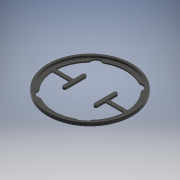
# Autodesk Inventor part: bumper_modified2
Saved by Autodesk Inventor 2017 SP1 (Build 210196100, 196)
## iProperties
Created: 2016-07-25
Part Number: bumper_modified2
Material: Plastique ABS
Document SubType Name: Modeling
Designer: tmonglon
Density: 1.06 g/cm^3
Appearance: Lisse - Noir
Author: tmonglon
Autodesk Inventor part; units mm, degrees
ref_plane "YZ Plane" through (0, 0, 0) normal (1, 0, 0) x (0, 1, 0)
ref_plane "XZ Plane" through (0, 0, 0) normal (0, 1, 0) x (-1, 0, 0)
ref_plane "XY Plane" through (0, 0, 0) normal (0, 0, 1) x (1, 0, 0)
sketch "Esquisse1" plane through (0, 0, 0) normal (0, 0, 1) x (1, 0, 0)
  circle A0 centre (0, 0) radius 63
  circle A1 centre (0, 0) radius 60
  circle A2 centre (0, 0) radius 54
  line L0 (-25.9421, 2.5) -> (-53.9421, 2.5)
  line L1 (-25.9421, -2.5) -> (-53.9421, -2.5)
  line L2 (-20.9421, 0) -> (-20.9421, 14.5)
  line L3 (-25.9421, 14.5) -> (-25.9421, 2.5)
  line L4 (-20.9421, 0) -> (-20.9421, -14.5)
  line L5 (-25.9421, -14.5) -> (-25.9421, 2.5)
  arc A3 (-25.9421, -14.5) -> (-20.9421, -14.5) centre (-23.4421, -14.5) ccw
  arc A4 (-20.9421, 14.5) -> (-25.9421, 14.5) centre (-23.4421, 14.5) ccw
  line L6 (0, 0) -> (0, 11.8583)
  line L7 (25.9421, 2.5) -> (53.9421, 2.5)
  line L8 (25.9421, -2.5) -> (53.9421, -2.5)
  line L9 (20.9421, 0) -> (20.9421, 14.5)
  line L10 (25.9421, 14.5) -> (25.9421, 2.5)
  line L11 (20.9421, 0) -> (20.9421, -14.5)
  line L12 (25.9421, -14.5) -> (25.9421, 14.5)
  arc A5 (20.9421, -14.5) -> (25.9421, -14.5) centre (23.4421, -14.5) ccw
  arc A6 (25.9421, 14.5) -> (20.9421, 14.5) centre (23.4421, 14.5) ccw
  line L13 (25.9421, 2.5) -> (56.5559, 2.5)
  line L14 (56.5559, 2.5) -> (56.5559, -2.5)
  line L15 (56.5559, -2.5) -> (25.9421, -2.5)
  line L16 (25.9421, -2.5) -> (25.9421, 2.5)
  dimension "d0" = 126
  dimension "d1" = 120
  dimension "d2" = 108
  dimension "d3" = 28
  dimension "d6" = 14.5
  dimension "d8" = 5
  constraints: 34 end point, 11 point on circle, 11 symmetric about line, 7 centre point, 6 point on line, 4 parallel, 1 coincident, 1 horizontal, 1 perpendicular, 1 vertical, 2 other
  measures "d0" diameter of A0
  measures "d1" diameter of A1
  measures "d2" diameter of A2
  measures "d3" distance of L0.start L0.end
  measures "d6" distance of L2.start L2.end
  measures "d8" distance of L4.end L5.start
extrude "Extrusion1" add sketch "Esquisse1" along normal blind 5 contours A0
extrude "Extrusion2" add sketch "Esquisse1" along normal blind 1.7 contours A1 | A2 L8 L12 L7 | A2 L13 L14 L15 | L0 L5 L1 A2
sketch "Esquisse3" plane through (0, 0, 0) normal (0, 0, -1) x (-1, 0, 0)
  line L0 (20.9421, 0) -> (20.9421, 14.5) projected
  line L1 (20.9421, 0) -> (20.9421, -14.5) projected
  arc A0 (20.9421, -14.5) -> (25.9421, -14.5) centre (23.4421, -14.5) ccw projected
  line L2 (25.9421, -14.5) -> (25.9421, 2.5) projected
  line L3 (25.9421, 14.5) -> (25.9421, 2.5) projected
  arc A1 (25.9421, 14.5) -> (20.9421, 14.5) centre (23.4421, 14.5) ccw projected
  arc A2 (-20.9421, 14.5) -> (-25.9421, 14.5) centre (-23.4421, 14.5) ccw projected
  line L4 (-25.9421, 14.5) -> (-25.9421, 2.5) projected
  line L5 (-25.9421, -14.5) -> (-25.9421, 14.5) projected
  arc A3 (-25.9421, -14.5) -> (-20.9421, -14.5) centre (-23.4421, -14.5) ccw projected
  line L6 (-20.9421, 0) -> (-20.9421, -14.5) projected
  line L7 (-20.9421, 0) -> (-20.9421, 14.5) projected
  point P0 (0, 0)
extrude "Extrusion3" add sketch "Esquisse3" against normal blind 3
fillet "Congé1" radius 1 3 edges at (25.9421, 0, 1.7) (25.9421, -2.5, 0.85) (25.9421, 2.5, 0.85)
fillet "Congé2" radius 1 3 edges at (-25.9421, 0, 1.7) (-25.9421, -2.5, 0.85) (-25.9421, 2.5, 0.85)
fillet "Congé3" radius 1 4 edges at (53.9421, 2.5, 0.85) (53.9421, -2.5, 0.85) (-53.9421, 2.5, 0.85) (-53.9421, -2.5, 0.85)
sketch "Esquisse4" plane through (0, 0, 0) normal (0, 0, -1) x (-1, 0, 0)
  arc A0 (53.8821, 3.566) -> (-53.8821, 3.566) centre (0, 0) ccw projected
  arc A1 (-53.8821, -3.566) -> (53.8821, -3.566) centre (0, 0) ccw projected
  arc A2 (53.8821, 3.566) -> (-53.8821, 3.566) centre (0, 0) ccw projected
  arc A3 (52.8843, 2.5) -> (53.8821, 3.566) centre (52.8843, 3.5) ccw projected
  line L0 (52.8843, 2.5) -> (26.9421, 2.5) projected
  arc A4 (25.9421, 3.5) -> (26.9421, 2.5) centre (26.9421, 3.5) ccw projected
  line L1 (25.9421, 3.5) -> (25.9421, 14.5) projected
  arc A5 (25.9421, 14.5) -> (20.9421, 14.5) centre (23.4421, 14.5) ccw projected
  line L2 (20.9421, 14.5) -> (20.9421, -14.5) projected
  arc A6 (20.9421, -14.5) -> (25.9421, -14.5) centre (23.4421, -14.5) ccw projected
  line L3 (25.9421, -14.5) -> (25.9421, -3.5) projected
  arc A7 (26.9421, -2.5) -> (25.9421, -3.5) centre (26.9421, -3.5) ccw projected
  line L4 (26.9421, -2.5) -> (52.8843, -2.5) projected
  arc A8 (53.8821, -3.566) -> (52.8843, -2.5) centre (52.8843, -3.5) ccw projected
  arc A9 (-53.8821, -3.566) -> (53.8821, -3.566) centre (0, 0) ccw projected
  arc A10 (-52.8843, -2.5) -> (-53.8821, -3.566) centre (-52.8843, -3.5) ccw projected
  line L5 (-26.9421, -2.5) -> (-52.8843, -2.5) projected
  arc A11 (-25.9421, -3.5) -> (-26.9421, -2.5) centre (-26.9421, -3.5) ccw projected
  line L6 (-25.9421, -3.5) -> (-25.9421, -14.5) projected
  arc A12 (-25.9421, -14.5) -> (-20.9421, -14.5) centre (-23.4421, -14.5) ccw projected
  line L7 (-20.9421, -14.5) -> (-20.9421, 14.5) projected
  arc A13 (-20.9421, 14.5) -> (-25.9421, 14.5) centre (-23.4421, 14.5) ccw projected
  line L8 (-25.9421, 14.5) -> (-25.9421, 3.5) projected
  arc A14 (-26.9421, 2.5) -> (-25.9421, 3.5) centre (-26.9421, 3.5) ccw projected
  line L9 (-52.8843, 2.5) -> (-26.9421, 2.5) projected
  arc A15 (-53.8821, 3.566) -> (-52.8843, 2.5) centre (-52.8843, 3.5) ccw projected
  circle A16 centre (0, 0) radius 63 projected
  line L10 (32.9786, 41.9728) -> (-33, 41.9728)
  line L11 (-33, 41.9728) -> (-33, -42)
  line L12 (-33, -42) -> (32.9786, -42)
  line L13 (32.9786, -42) -> (32.9786, 41.9728)
  line L14 (32.9786, 32.8) -> (-33, 32.8)
  line L15 (32.9786, -32.8) -> (-33, -32.8)
  line L16 (-33.3624, -42.4612) -> (38.9228, 49.5381)
  line L17 (33.3492, -42.4716) -> (-38.936, 49.5277)
  line L18 (-33.2831, 42.3332) -> (-36.4284, 39.8619)
  line L19 (-33.2831, 42.3332) -> (-30.1379, 44.8045)
  arc A17 (-30.1379, 44.8045) -> (-36.4284, 39.8619) centre (-32.5624, 41.4158) ccw
  line L20 (33.2707, 42.3445) -> (30.1254, 44.8158)
  line L21 (33.2707, 42.3445) -> (36.416, 39.8733)
  line L22 (33.2831, -42.3332) -> (36.4284, -39.8619)
  line L23 (33.2831, -42.3332) -> (30.1379, -44.8045)
  arc A18 (30.1379, -44.8045) -> (36.4284, -39.8619) centre (32.5624, -41.4158) ccw
  arc A19 (36.416, 39.8733) -> (30.1254, 44.8158) centre (32.5499, 41.4272) ccw
  line L24 (-33.2707, -42.3445) -> (-36.416, -39.8733)
  arc A20 (-36.416, -39.8733) -> (-30.1254, -44.8158) centre (-32.5499, -41.4272) ccw
  line L25 (-33.2707, -42.3445) -> (-30.1254, -44.8158)
  arc A21 (-53.8821, -3.566) -> (53.8821, -3.566) centre (0, 0) ccw projected
  line L26 (-38.5851, -37.7782) -> (-27.5766, -46.4277)
  arc A22 (-38.5851, -37.7782) -> (-27.5766, -46.4277) centre (-31.4173, -39.9857) ccw
  line L27 (-38.5969, 37.7661) -> (-27.5885, 46.4156)
  arc A23 (-27.5885, 46.4156) -> (-38.5969, 37.7661) centre (-31.4292, 39.9736) ccw
  line L28 (27.5621, -46.4363) -> (38.5705, -37.7868)
  arc A24 (27.5621, -46.4363) -> (38.5705, -37.7868) centre (31.4028, -39.9943) ccw
  line L29 (27.5766, 46.4277) -> (38.5851, 37.7782)
  arc A25 (38.5851, 37.7782) -> (27.5766, 46.4277) centre (31.4173, 39.9857) ccw
  point P0 (-35.1366, 44.6921)
  point P1 (35.1242, 44.7035)
  point P2 (33, -41.9728)
  point P3 (35.1366, -44.6921)
  point P4 (-32.9786, -41.9728)
  point P5 (-35.1242, -44.7035)
  point P6 (-38.9228, -49.5381)
  dimension "d42" = 33
  dimension "d43" = 42
  dimension "d44" = 4
  dimension "d45" = 4
  dimension "d46" = 3
  dimension "d47" = 65.9786
  dimension "d48" = 83.9728
  dimension "d53" = 4
  dimension "d54" = 4
  dimension "d55" = 3
  dimension "d58" = 360
  dimension "d62" = 360
  dimension "d80" = 7
  dimension "d81" = 14
  dimension "d82" = 7.5
  dimension "d83" = 14
  dimension "d84" = 7
  dimension "d85" = 7.5
  dimension "d86" = 14
  dimension "d87" = 7
  dimension "d88" = 7.5
  dimension "d89" = 14
  dimension "d90" = 7
  dimension "d91" = 7.5
  constraints: 40 end point, 30 point on circle, 12 point on line, 8 centre point, 7 perpendicular, 6 parallel, 1 horizontal, 40 other
  measures "d42" distance from line of point (0, 0) L11
  measures "d43" distance from line of L12 point (0, 0)
  measures "d44" distance of L18.start L18.end
  measures "d45" distance of L18.start L19.end
  measures "d46" distance of L18.start point (-35.137, 44.692)
  measures "d47" distance of L11.end L12.end
  measures "d48" distance of L10.end L11.end
  measures "d53" distance of L20.start L20.end
  measures "d54" distance of L20.start L21.end
  measures "d55" distance of L20.start point (35.124, 44.703)
  measures "d80" distance from line of L26.end L16
  measures "d81" distance of L26.start L26.end
  measures "d82" radius of A22
  measures "d83" distance of L27.start L27.end
  measures "d84" distance from line of L17 L27.start
  measures "d85" radius of A23
  measures "d86" distance of L28.start L28.end
  measures "d87" distance from line of L17 L28.start
  measures "d88" radius of A24
  measures "d89" distance of L29.start L29.end
  measures "d90" distance from line of L16 L29.end
  measures "d91" radius of A25
extrude "Extrusion4" cut sketch "Esquisse4" against normal blind 10 contours L25 A1 L16 | L16 A1 L24 | A20 A1
extrude "Extrusion5" cut sketch "Esquisse4" against normal blind 10 contours L18 A0 L17 | A0 A17 L17 picked at (-34.5217, 42.711)
extrude "Extrusion6" cut sketch "Esquisse4" against normal blind 10 contours L19 L17 A0 | A0 L17 A17 picked at (-33.3576, 43.626)
extrude "Extrusion7" cut sketch "Esquisse4" against normal blind 10 contours L21 L16 A0 | A0 L16 A19 picked at (34.5088, 42.7218)
extrude "Extrusion8" cut sketch "Esquisse4" against normal blind 10 contours A18 A1 | A1 L17 L23 L22 | L17 A1 L23
extrude "Extrusion9" cut sketch "Esquisse4" against normal blind 10 contours L16 L20 A0 | A0 A19 L16 picked at (33.3443, 43.6367)
fillet "Congé4" radius 4 6 edges at (36.416, -39.8733, 0.85) (30.1254, -44.8158, 0.85) (36.4284, 39.8619, 0.85) (-36.416, 39.8733, 0.85) (-30.14, -44.806, 0.85) (-36.4284, -39.8619, 0.85)
extrude "Extrusion10" cut sketch "Esquisse4" against normal blind 10 contours A24 A1 A18 | A1 L22 L23 L17 L28 A24 | L17 L23 A1 L28
extrude "Extrusion11" cut sketch "Esquisse4" against normal blind 10 contours L29 L16 L21 A0 | A0 A19 L16 A25 | L29 A0 L20 L16 | L16 A19 A0 A25
extrude "Extrusion12" cut sketch "Esquisse4" against normal blind 10 contours A23 L27 L17 L19 A0 | A0 A17 L17 A23 | L27 A0 L18 L17 | L17 A17 A0 A23
extrude "Extrusion13" cut sketch "Esquisse4" against normal blind 10 contours L26 A1 L25 L16 | L16 L24 A1 L26 | A22 A1 A20
fillet "Congé5" radius 4 8 edges at (38.5851, -37.7782, 0.85) (27.5766, -46.4277, 0.85) (-27.5621, -46.4363, 0.85) (-38.572, -37.7916, 0.85) (27.5927, 46.4181, 0.85) (38.5969, 37.7661, 0.85) (-38.5851, 37.7782, 0.85) (-27.5766, 46.4277, 0.85)
equation "\"d80\" = 0.5 * d81"
equation "\"d90\" = 0.5 * d89"
